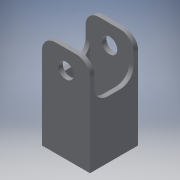
# Autodesk Inventor part: body-braket
Saved by Autodesk Inventor 2018.2 (Build 222227000, 227)
## iProperties
Created: 2018-05-02
Part Number: body-braket
Material: 一般
Document SubType Name: Modeling
Designer: ku_sk
Density: 1 g/cm^3
Appearance: 既定
Author: ku_sk
Autodesk Inventor part; units mm, degrees
ref_plane "YZ Plane" through (0, 0, 0) normal (1, 0, 0) x (0, 1, 0)
ref_plane "XZ Plane" through (0, 0, 0) normal (0, 1, 0) x (-1, 0, 0)
ref_plane "XY Plane" through (0, 0, 0) normal (0, 0, 1) x (1, 0, 0)
sketch "スケッチ1" plane through (0, 0, 0) normal (0, 0, 1) x (1, 0, 0)
  line L0 (-12.5, 12.5) -> (12.5, 12.5)
  line L1 (12.5, 12.5) -> (12.5, -12.5)
  line L2 (12.5, -12.5) -> (-12.5, -12.5)
  line L3 (-12.5, -12.5) -> (-12.5, 12.5)
  line L4 (-12.5, 12.5) -> (12.5, -12.5) construction
  line L5 (12.5, 12.5) -> (-12.5, -12.5) construction
  point P0 (0, 0)
  dimension "d0" = 25
  dimension "d1" = 25
  constraints: 12 end point, 2 midpoint, 2 parallel, 1 horizontal, 1 perpendicular
  measures "d0" distance of L0.start L0.end
  measures "d1" distance of L2.end L0.start
extrude "押し出し1" add sketch "スケッチ1" along normal mid plane 50
shell "シェル1" thickness 2.3 removed faces 2 at (-4.1667, -4.1667, 25) at (-4.1667, -4.1667, -25)
sketch "スケッチ2" plane through (12.5, -12.5, 25) normal (1, 0, 0) x (0, 0, -1)
  line L0 (0, 22.7) -> (20, 22.7)
  line L1 (20, 22.7) -> (20, 2.3)
  line L2 (20, 2.3) -> (0, 2.3)
  line L3 (0, 2.3) -> (0, 22.7)
  line L4 (0, 22.7) -> (20, 2.3) construction
  line L5 (20, 22.7) -> (0, 2.3) construction
  line L6 (0, 0) -> (0, 25) projected
  point P0 (25, 12.5)
  point P1 (10, 12.5)
  dimension "d5" = 20
  constraints: 12 end point, 2 midpoint, 2 parallel, 1 collinear, 1 horizontal, 1 perpendicular
  measures "d5" distance of L0.start L0.end
extrude "押し出し2" cut sketch "スケッチ2" against normal through all
sketch "スケッチ3" plane through (-12.5, 12.5, 25) normal (0, 1, 0) x (1, 0, 0)
  circle A0 centre (12.5, 10) radius 4
  line L0 (25, 0) -> (0, 0) projected
  line L1 (0, 50) -> (0, 0) projected
  point P0 (12.5, 25)
  dimension "d8" = 8
  dimension "d9" = 10
  dimension "d10" = 12.5
  constraints: 1 centre point
  measures "d8" diameter of A0
  measures "d9" distance from line of L0 A0.centre
  measures "d10" distance from line of L1 A0.centre
extrude "押し出し3" cut sketch "スケッチ3" against normal through all
fillet "フィレット1" radius 7 8 edges at (12.5, -11.35, 25) (-12.5, -11.35, 25) (-12.5, 11.35, 25) (12.5, 11.35, 25) (11.35, 10.2, 5) (-11.35, 10.2, 5) (-11.35, -10.2, 5) (11.35, -10.2, 5)
equation "\"d1\" = d0"
